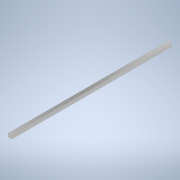
# Autodesk Inventor part: ロボットベース15x15_1
Saved by Autodesk Inventor 2020.3 (Build 243373000, 373)
## iProperties
Created: 2020-07-04
Part Number: ロボットベース15x15_1
Material: アルミニウム 6061
Document SubType Name: Modeling
Designer: totot
Density: 2.7 g/cm^3
Appearance: アルミニウム - フラット
Author: totot
Autodesk Inventor part; units mm, degrees
ref_plane "YZ Plane" through (0, 0, 0) normal (1, 0, 0) x (0, 1, 0)
ref_plane "XZ Plane" through (0, 0, 0) normal (0, 1, 0) x (-1, 0, 0)
ref_plane "XY Plane" through (0, 0, 0) normal (0, 0, 1) x (1, 0, 0)
sketch "スケッチ1" plane through (0, 0, 0) normal (0, 0, 1) x (1, 0, 0)
  line L0 (0, 0) -> (-15, 0)
  line L1 (-15, 0) -> (-15, -15)
  line L2 (-15, -15) -> (0, -15)
  line L3 (0, -15) -> (0, 0)
  line L4 (-13.8, -1.2) -> (-1.2, -1.2)
  line L5 (-1.2, -1.2) -> (-1.2, -13.8)
  line L6 (-1.2, -13.8) -> (-13.8, -13.8)
  line L7 (-13.8, -13.8) -> (-13.8, -1.2)
  dimension "d0" = 15
  dimension "d1" = 15
  dimension "d2" = 1.2
  dimension "d3" = 1.2
  dimension "d4" = 1.2
  dimension "d5" = 1.2
  constraints: 16 end point, 4 parallel, 2 horizontal, 2 perpendicular
  measures "d0" distance of L2.end L1.end
  measures "d1" distance of L1.end L0.end
  measures "d2" distance between parallel lines of L1 L7
  measures "d3" distance between parallel lines of L4 L0
  measures "d4" distance between parallel lines of L2 L6
  measures "d5" distance between parallel lines of L5 L3
extrude "押し出し1" add sketch "スケッチ1" along normal blind 655
sketch "スケッチ2" plane through (0, -15, 0) normal (1, 0, 0) x (0, 0, -1)
  line L0 (-655, 0) -> (-655, 15) projected
  line L1 (0, 15) -> (-655, 15) projected
  line L2 (0, 0) -> (0, 15) projected
  point P0 (-7.5, 7.5)
  point P1 (-647.5, 7.5)
  dimension "d8" = 7.5
  dimension "d9" = 7.5
  dimension "d10" = 7.5
  dimension "d11" = 7.5
  measures "d8" distance from line of point (-647.5, 7.5) L0
  measures "d9" distance from line of point (-647.5, 7.5) L1
  measures "d10" distance from line of point (-7.5, 7.5) L1
  measures "d11" distance from line of point (-7.5, 7.5) L2
hole "穴1" at (0, -7.5, 7.5) at (0, -7.5, 647.5) direction (-1, 0, 0) diameter 5 end through all
sketch "スケッチ3" plane through (-15, -15, 0) normal (-1, 0, 0) x (0, 0, 1)
  line L0 (0, 0) -> (655, 0) projected
  circle A0 centre (7.5, 7.5) radius 2.5 projected
  circle A1 centre (647.5, 7.5) radius 2.5 projected
  point P0 (0, 15)
  point P1 (22.5, 7.5)
  point P2 (632.5, 7.5)
  dimension "d19" = 7.5
  dimension "d20" = 15
  dimension "d21" = 7.5
  dimension "d22" = 15
  measures "d19" distance from line of point (22.5, 7.5) L0
  measures "d20" distance of point (22.5, 7.5) A0.centre
  measures "d21" distance from line of L0 point (632.5, 7.5)
  measures "d22" distance of point (632.5, 7.5) A1.centre
hole "穴2" at (-15, -7.5, 22.5) at (-15, -7.5, 632.5) direction (1, 0, 0) diameter 3 depth 5 tip angle 118
sketch "スケッチ4" plane through (-1.2, -13.8, 0) normal (-1, 0, 0) x (0, 0, 1)
  circle A0 centre (22.5, 6.3) radius 1.5 projected
  circle A1 centre (632.5, 6.3) radius 1.5 projected
  point P0 (0, 13.8)
  constraints: 2 coincident
hole "穴3" at (-1.2, -7.5, 22.5) at (-1.2, -7.5, 632.5) direction (1, 0, 0) diameter 6 end through all
sketch "スケッチ6" plane through (-15, 0, 0) normal (0, 1, 0) x (1, 0, 0)
  line L0 (15, -655) -> (0, -655) projected
  line L1 (15, 0) -> (15, -655) projected
  line L2 (15, 0) -> (0, 0) projected
  point P0 (7.5, -37.5)
  point P1 (7.5, -617.5)
  dimension "d37" = 37.5
  dimension "d38" = 7.5
  dimension "d39" = 7.5
  dimension "d40" = 37.5
  measures "d37" distance from line of point (7.5, -617.5) L0
  measures "d38" distance from line of point (7.5, -617.5) L1
  measures "d39" distance from line of point (7.5, -37.5) L1
  measures "d40" distance from line of point (7.5, -37.5) L2
hole "穴4" at (-7.5, 0, 37.5) at (-7.5, 0, 617.5) direction (0, -1, 0) diameter 3 end through all
sketch "スケッチ7" plane through (-15, -15, 0) normal (-1, 0, 0) x (0, 0, 1)
  line L0 (0, 15) -> (655, 15) projected
  line L1 (0, 15) -> (0, 0) projected
  point P0 (327.5, 7.5)
  dimension "d59" = 655
  dimension "d60" = 327.5
  dimension "d61" = 7.5
  measures "d59" distance of L0.start L0.end
  measures "d60" distance from line of point (327.5, 7.5) L1
  measures "d61" distance from line of point (327.5, 7.5) L0
hole "穴5" at (-15, -7.5, 327.5) direction (1, 0, 0) diameter 5 end through all
sketch "スケッチ8" plane through (-15, -15, 0) normal (-1, 0, 0) x (0, 0, 1)
  line L0 (0, 15) -> (655, 15) projected
  circle A0 centre (327.5, 7.5) radius 2.5 projected
  point P0 (277, 7.5)
  point P1 (378, 7.5)
  dimension "d62" = 7.5
  dimension "d63" = 7.5
  dimension "d64" = 101
  dimension "d65" = 50.5
  measures "d62" distance from line of point (277, 7.5) L0
  measures "d63" distance from line of point (378, 7.5) L0
  measures "d64" distance of point (378, 7.5) point (277, 7.5)
  measures "d65" distance of point (277, 7.5) A0.centre
hole "穴6" at (-15, -7.5, 277) at (-15, -7.5, 378) direction (1, 0, 0) diameter 3 end through all
sketch "スケッチ9" plane through (-15, 0, 0) normal (0, 1, 0) x (1, 0, 0)
  line L0 (15, 0) -> (15, -655) projected
  line L1 (15, 0) -> (0, 0) projected
  point P0 (7.5, -292)
  point P1 (7.5, -363)
  dimension "d73" = 7.5
  dimension "d74" = 7.5
  dimension "d75" = 71
  dimension "d76" = 655
  dimension "d77" = 292
  measures "d73" distance from line of point (7.5, -292) L0
  measures "d74" distance from line of point (7.5, -363) L0
  measures "d75" distance of point (7.5, -292) point (7.5, -363)
  measures "d76" distance of L0.start L0.end
  measures "d77" distance from line of point (7.5, -292) L1
hole "穴7" at (-7.5, 0, 292) at (-7.5, 0, 363) direction (0, -1, 0) diameter 3 end through all
equation "\"d3\" = d2"
equation "\"d4\" = d3"
equation "\"d5\" = d2"
equation "\"d9\" = d8"
equation "\"d11\" = d10"
equation "\"d60\" = 0.5 * d59"
equation "\"d61\" = d57"
equation "\"d63\" = d62"
equation "\"d74\" = d73"
equation "\"d77\" = -0.5 * d75 + 0.5 * d76"
equation "\"d57\" = 7.5"
